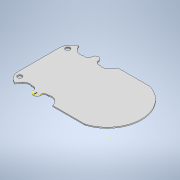
# Autodesk Inventor part: Onderplaat-v1
Saved by Autodesk Inventor 2022 (Build 260153000, 153)
## iProperties
Created: 2021-11-25
Part Number: Onderplaat-v1
Material: Generic
Document SubType Name: Modeling
Designer: keemi
Density: 1 g/cm^3
Appearance: Default
Author: keemi
Autodesk Inventor part; units mm, degrees
ref_plane "YZ Plane" through (0, 0, 0) normal (1, 0, 0) x (0, 1, 0)
ref_plane "XZ Plane" through (0, 0, 0) normal (0, 1, 0) x (-1, 0, 0)
ref_plane "XY Plane" through (0, 0, 0) normal (0, 0, 1) x (1, 0, 0)
sketch "Sketch1" plane through (0, 0, 0) normal (0, 1, 0) x (-1, 0, 0)
  line L0 (300, -35) -> (300, -155)
  line L1 (220, -190) -> (220, -190)
  line L2 (255, -180) -> (255, -180)
  line L3 (245, -170) -> (240, -170)
  line L4 (230, -180) -> (230, -180)
  line L5 (220, -190) -> (220, -190)
  line L6 (185, -180) -> (185, -180)
  line L7 (195, -170) -> (200, -170)
  line L8 (210, -180) -> (210, -180)
  arc A0 (255, -172) -> (253, -170) centre (253, -172) ccw
  arc A1 (255, -180) -> (245, -170) centre (245, -180) ccw
  arc A2 (240, -170) -> (230, -180) centre (240, -180) ccw
  arc A3 (210, -180) -> (220, -190) centre (220, -180) ccw
  arc A4 (220, -190) -> (230, -180) centre (220, -180) ccw
  arc A5 (210, -180) -> (200, -170) centre (200, -180) ccw
  arc A6 (195, -170) -> (185, -180) centre (195, -180) ccw
  arc A7 (175, -190) -> (185, -180) centre (175, -180) ccw
  line L9 (265, -190) -> (265, -190)
  arc A8 (255, -180) -> (265, -190) centre (265, -180) ccw
  line L10 (220, 0) -> (220, 0)
  line L11 (255, -10) -> (255, -10)
  line L12 (245, -20) -> (240, -20)
  line L13 (230, -10) -> (230, -10)
  line L14 (220, 0) -> (220, 0)
  line L15 (185, -10) -> (185, -10)
  line L16 (195, -20) -> (200, -20)
  line L17 (210, -10) -> (210, -10)
  arc A9 (253, -20) -> (255, -18) centre (253, -18) ccw
  arc A10 (245, -20) -> (255, -10) centre (245, -10) ccw
  arc A11 (230, -10) -> (240, -20) centre (240, -10) ccw
  arc A12 (220, 0) -> (210, -10) centre (220, -10) ccw
  arc A13 (230, -10) -> (220, 0) centre (220, -10) ccw
  arc A14 (200, -20) -> (210, -10) centre (200, -10) ccw
  arc A15 (185, -10) -> (195, -20) centre (195, -10) ccw
  arc A16 (185, -10) -> (175, 0) centre (175, -10) ccw
  line L18 (265, 0) -> (265, 0)
  arc A17 (265, 0) -> (255, -10) centre (265, -10) ccw
  arc A18 (265, -190) -> (300, -155) centre (265, -155) ccw
  arc A19 (300, -35) -> (265, 0) centre (265, -35) ccw
  line L19 (175, 0) -> (365, 0) construction
  arc A20 (70, 0) -> (70, -190) centre (99.4643, -95) ccw
  line L20 (175, 0) -> (70, 0)
  line L21 (175, -190) -> (70, -190)
  point P0 (0, 0)
  point P1 (300, -190)
  point P2 (300, 0)
  point P3 (255, -170)
  point P4 (255, -190)
  point P5 (230, -170)
  point P6 (185, -170)
  point P7 (210, -170)
  point P8 (255, -20)
  point P9 (255, 0)
  point P10 (230, -20)
  point P11 (185, -20)
  point P12 (210, -20)
  point P13 (210, -10)
  dimension "d1" = 190
  dimension "d2" = 80
  dimension "d4" = 25
  dimension "d5" = 20
  dimension "d7" = 25
  dimension "d9" = 2
  dimension "d10" = 10
  dimension "d11" = 10
  dimension "d12" = 35
  constraints: 44 end point, 42 point on circle, 28 point on line, 21 centre point, 21 tangent, 7 equal radius, 3 horizontal, 2 parallel, 1 perpendicular
  measures "d1" distance of point (300, 0) point (300, -190)
  measures "d2" distance of point (300, -190) L1.end
  measures "d4" distance of point (230, -170) point (255, -170)
  measures "d5" distance of point (255, -170) point (255, -190)
  measures "d7" distance of point (185, -170) point (210, -170)
  measures "d9" radius of A0
  measures "d10" radius of A1
  measures "d11" radius of A8
  measures "d12" radius of A18
extrude "Extrusion1" add sketch "Sketch1" along normal blind 3
sketch "Sketch2" plane through (0, 3, 0) normal (0, 1, 0) x (1, 0, 0)
  arc A0 (-230, 10) -> (-210, 10) centre (-220, 10) ccw projected
  line L0 (-220, 0) -> (-220, 10)
  point P0 (0, 0)
  constraints: 2 end point, 1 point on circle, 1 vertical
sketch "Sketch3" plane through (0, 3, 0) normal (0, 1, 0) x (1, 0, 0)
  arc A0 (-245, 20) -> (-255, 10) centre (-245, 10) ccw projected
  arc A1 (-300, 35) -> (-265, 0) centre (-265, 35) ccw projected
  arc A2 (-245, 20) -> (-276.1181, 1.8128) centre (-249.7009, -7.6718) ccw
  line L0 (-276.1181, 1.8128) -> (-248.5566, -2.5367)
  line L1 (-248.5566, -2.5367) -> (-245, 20)
  arc A3 (-230, 10) -> (-210, 10) centre (-220, 10) ccw projected
  line L2 (-220, 0) -> (-220, 190)
  arc A4 (-210, 180) -> (-230, 180) centre (-220, 180) ccw projected
  arc A5 (-163.8819, 1.8128) -> (-195, 20) centre (-190.2991, -7.6718) ccw
  line L3 (-191.4434, -2.5367) -> (-195, 20)
  line L4 (-163.8819, 1.8128) -> (-191.4434, -2.5367)
  line L5 (-220, 95) -> (-300, 95)
  line L6 (-300, 155) -> (-300, 35) projected
  arc A6 (-276.1181, 188.1872) -> (-245, 170) centre (-249.7009, 197.6718) ccw
  line L7 (-276.1181, 188.1872) -> (-248.5566, 192.5367)
  line L8 (-248.5566, 192.5367) -> (-245, 170)
  arc A7 (-195, 170) -> (-163.8819, 188.1872) centre (-190.2991, 197.6718) ccw
  line L9 (-191.4434, 192.5367) -> (-195, 170)
  line L10 (-163.8819, 188.1872) -> (-191.4434, 192.5367)
  point P0 (0, 0)
  constraints: 20 end point, 12 symmetric about line, 11 point on circle, 4 centre point, 2 midpoint, 1 perpendicular, 1 vertical, 3 other
extrude "Extrusion2" cut sketch "Sketch3" against normal blind 10
sketch "Sketch4" plane through (0, 3, 0) normal (0, 1, 0) x (1, 0, 0)
  line L0 (-300, 155) -> (-300, 35) projected
  line L1 (-300, 35) -> (-285, 35)
  line L2 (-285, 35) -> (-285, 25)
  circle A0 centre (-285, 25) radius 6.5
  line L3 (-300, 155) -> (-285, 155)
  line L4 (-300, 155) -> (-285, 155) construction
  line L5 (-285, 155) -> (-285, 165)
  circle A1 centre (-285, 165) radius 6.5
  point P0 (0, 0)
  dimension "d19" = 15
  dimension "d20" = 10
  dimension "d21" = 13
  dimension "d22" = 15
  dimension "d24" = 10
  dimension "d25" = 13
  constraints: 10 end point, 3 horizontal, 2 centre point, 2 coincident, 2 perpendicular, 1 collinear
  measures "d19" distance of L0.end L1.end
  measures "d20" distance of L1.end L2.end
  measures "d21" diameter of A0
  measures "d22" distance of L0.start L3.end
  measures "d24" distance of L4.end L5.end
  measures "d25" diameter of A1
extrude "Extrusion3" cut sketch "Sketch4" against normal blind 10
sketch "Sketch5" plane through (0, 3, 0) normal (0, 1, 0) x (1, 0, 0)
  line L0 (-175.3338, 0.0056) -> (-163.8819, 1.8128) projected
  line L1 (-163.8819, 1.8128) -> (-179.2892, 1.8128)
  line L2 (-179.2892, 1.8128) -> (-179.2892, -4.2644)
  line L3 (-179.2892, -4.2644) -> (-163.8819, -4.2644)
  line L4 (-163.8819, -4.2644) -> (-163.8819, 1.8128)
  arc A0 (-300, 35) -> (-276.1181, 1.8128) centre (-265, 35) ccw projected
  line L5 (-276.1181, 1.8128) -> (-262.1006, 1.8128)
  line L6 (-262.1006, 1.8128) -> (-262.1006, -4.2644)
  line L7 (-262.1006, -4.2644) -> (-276.1181, -4.2644)
  line L8 (-276.1181, -4.2644) -> (-276.1181, 1.8128)
  line L9 (-163.8819, 188.1872) -> (-175.3338, 189.9944) projected
  line L10 (-163.8819, 188.1872) -> (-177.2047, 188.1872)
  line L11 (-177.2047, 188.1872) -> (-177.2047, 195.4302)
  line L12 (-177.2047, 195.4302) -> (-163.8819, 195.4302)
  line L13 (-163.8819, 195.4302) -> (-163.8819, 188.1872)
  arc A1 (-276.1181, 188.1872) -> (-245, 170) centre (-249.7009, 197.6718) ccw projected
  line L14 (-276.1181, 188.1872) -> (-262.1006, 188.1872)
  line L15 (-262.1006, 188.1872) -> (-262.1006, 191.8087)
  line L16 (-262.1006, 191.8087) -> (-276.1181, 191.8087)
  line L17 (-276.1181, 191.8087) -> (-276.1181, 188.1872)
  point P0 (0, 0)
  constraints: 32 end point, 8 parallel, 4 horizontal, 4 perpendicular, 2 point on line
extrude "Extrusion4" cut sketch "Sketch5" against normal blind 10
sketch "Sketch6" plane through (0, 3, 0) normal (0, 1, 0) x (1, 0, 0)
  arc A0 (-163.8819, 1.8128) -> (-195, 20) centre (-190.2991, -7.6718) ccw projected
  line L0 (-195, 20) -> (-173.6747, 14.9436)
  line L1 (-173.6747, 14.9436) -> (-195, 20)
  line L2 (-200, 20) -> (-195, 20) projected
  arc A1 (-173.6747, 14.9436) -> (-195, 20) centre (-187.6449, 3.5225) ccw
  arc A2 (-230, 10) -> (-210, 10) centre (-220, 10) ccw projected
  line L3 (-220, 0) -> (-220, 190)
  arc A3 (-210, 180) -> (-230, 180) centre (-220, 180) ccw projected
  line L4 (-300, 155) -> (-300, 35) projected
  line L5 (-300, 95) -> (0, 95)
  arc A4 (-245, 20) -> (-276.1181, 1.8128) centre (-249.7009, -7.6718) ccw
  line L6 (-245, 20) -> (-266.3253, 14.9436)
  line L7 (-266.3253, 14.9436) -> (-245, 20)
  arc A5 (-245, 20) -> (-266.3253, 14.9436) centre (-252.3551, 3.5225) ccw
  arc A6 (-195, 170) -> (-163.8819, 188.1872) centre (-190.2991, 197.6718) ccw
  line L8 (-195, 170) -> (-173.6747, 175.0564)
  line L9 (-173.6747, 175.0564) -> (-195, 170)
  line L10 (-200, 170) -> (-195, 170)
  arc A7 (-195, 170) -> (-173.6747, 175.0564) centre (-187.6449, 186.4775) ccw
  arc A8 (-210, 180) -> (-230, 180) centre (-220, 180) ccw
  line L11 (-220, 190) -> (-220, 0)
  arc A9 (-276.1181, 188.1872) -> (-245, 170) centre (-249.7009, 197.6718) ccw
  line L12 (-245, 170) -> (-266.3253, 175.0564)
  line L13 (-266.3253, 175.0564) -> (-245, 170)
  arc A10 (-266.3253, 175.0564) -> (-245, 170) centre (-252.3551, 186.4775) ccw
  point P0 (0, 0)
  constraints: 24 end point, 23 point on circle, 19 symmetric about line, 8 centre point, 1 horizontal, 1 midpoint, 1 vertical, 7 other
extrude "Extrusion5" cut sketch "Sketch6" against normal blind 10 contours L0 A0 | A0 A1 | A4 A5 | A6 A7 | A9 A10
body "Solid1"
